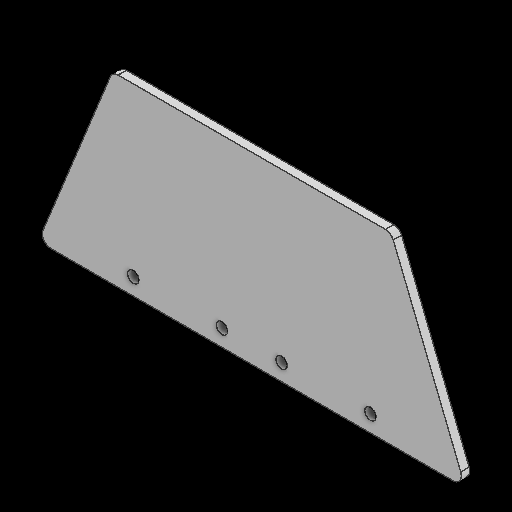
# Autodesk Inventor part: BreakerMount
Saved by Autodesk Inventor 2025.2 (Build 292293000, 293)
## iProperties
Created: 2025-11-18
Part Number: BreakerMount
Material: Generic
Document SubType Name: Sheet Metal
Designer: valer
Density: 1 g/cm^3
Sheet Metal Rule: Default
Appearance: Default
Author: valer
Autodesk Inventor part; units mm, degrees
ref_plane "YZ Plane" through (0, 0, 0) normal (1, 0, 0) x (0, 1, 0)
ref_plane "XZ Plane" through (0, 0, 0) normal (0, 1, 0) x (-1, 0, 0)
ref_plane "XY Plane" through (0, 0, 0) normal (0, 0, 1) x (1, 0, 0)
sketch "Base" plane through (0, 0, 0) normal (0, 0, 1) x (1, 0, 0)
  line L0 (0, 0) -> (70.3402, 0)
  line L1 (70.3402, 0) -> (115.4849, -88)
  line L2 (115.4849, -88) -> (0, -88)
  line L3 (0, -88) -> (0, 0) construction
  line L4 (0, 0) -> (-70.3402, 0)
  line L5 (-70.3402, 0) -> (-115.4849, -88)
  line L6 (-115.4849, -88) -> (0, -88)
  line L7 (-63.3831, 22.3248) -> (-182.4251, -209.7225) construction
  dimension "d1" = 88
  dimension "d3" = 4
  measures "d1" distance between parallel lines of L6 L4
  measures "d3" distance between parallel lines of L7 L5
extrude "Plate1" add sketch "Base" along normal blind 4
fillet "FilletsFeature" radius 6 4 edges at (-70.3402, 0, 2) (70.3402, 0, 2) (115.4849, -88, 2) (-115.4849, -88, 2)
sketch "BreakerMounts" plane through (0, 0, 0) normal (0, 0, -1) x (-1, 0, 0)
  circle A0 centre (56.75, -80) radius 2.75 projected
  circle A1 centre (14.25, -80) radius 2.75 projected
  circle A2 centre (-14.25, -80) radius 2.75 projected
  circle A3 centre (-56.75, -80) radius 2.75 projected
  point P0 (0, 0)
extrude "BreakerMountsFeature" cut sketch "BreakerMounts" against normal blind 4
sketch "FrameMounts" plane through (0, 0, 0) normal (0, 0, -1) x (-1, 0, 0)
  circle A0 centre (100.2396, -78) radius 3
  circle A1 centre (75.1349, -29.0638) radius 3
  line L0 (100.2396, -78) -> (75.1349, -29.0638) construction
  line L1 (72.0133, -3.2613) -> (111.0019, -79.2613) construction
  line L2 (105.6634, -88) -> (-105.6634, -88) projected
  line L3 (0, -105.6) -> (0, 17.6) construction
  circle A2 centre (-100.2396, -78) radius 3
  circle A3 centre (-75.1349, -29.0638) radius 3
  point P0 (0, 0)
  dimension "d6" = 6
  dimension "d7" = 6
  dimension "d8" = 10
  dimension "d9" = 9
  dimension "d10" = 55
  constraints: 4 centre point, 2 end point, 2 symmetric about line, 1 parallel, 2 other
  measures "d6" diameter of A0
  measures "d7" diameter of A1
  measures "d8" distance from line of L2 L0.start
  measures "d9" distance between parallel lines of L1 L0
  measures "d10" distance of L0.start L0.end
feature "FrameMountsFeature" [suppressed]
sketch "MatchProduction" plane through (0, 0, 4) normal (0, 0, 1) x (1, 0, 0)
  line L0 (0, -105.6) -> (0, 17.6) construction
  line L1 (-66.6748, 0) -> (66.6748, 0) projected
  line L2 (66.6748, 0) -> (102.2291, -88)
  line L3 (105.6634, -88) -> (-105.6634, -88) projected
  arc A0 (72.0133, -3.2613) -> (66.6748, 0) centre (66.6748, -6) ccw projected
  line L4 (72.0133, -3.2613) -> (111.0019, -79.2613) projected
  arc A1 (105.6634, -88) -> (111.0019, -79.2613) centre (105.6634, -82) ccw projected
  arc A2 (-111.0019, -79.2613) -> (-105.6634, -88) centre (-105.6634, -82) ccw projected
  line L5 (-111.0019, -79.2613) -> (-72.0133, -3.2613) projected
  arc A3 (-66.6748, 0) -> (-72.0133, -3.2613) centre (-66.6748, -6) ccw projected
  line L6 (-66.6748, 0) -> (-102.2291, -88)
  point P0 (0, 0)
  dimension "d13" = 68
  constraints: 4 end point, 1 point on line, 1 symmetric about line
  measures "d13" angle of L3 L2
extrude "MatchProductionFeature" cut sketch "MatchProduction" against normal blind 4 contours L6 L3 A2 L5 A3 | A0 L4 A1 L3 L2
fillet "Fillet2" radius 4 4 edges at (-102.2291, -88, 2) (102.2291, -88, 2) (66.6748, 0, 2) (-66.6748, 0, 2)
equation "\"d4\" = Thickness"
equation "\"d11\" = Thickness"
equation "\"d14\" = Thickness"
equation "\"d0\" = Thickness"
equation "\"BendRadius\" = Thickness"
equation "\"BendReliefWidth\" = Thickness"
equation "\"BendReliefDepth\" = 0.5 * Thickness"
equation "\"CornerReliefSize\" = 4 * Thickness"
equation "\"MinimumRemnant\" = 2 * Thickness"
equation "\"TransitionRadius\" = BendRadius"
equation "\"JacobiRadiusSize\" = BendRadius"
equation "\"GapSize\" = Thickness"
equation "\"Thickness\" = 4"
body "Solid1"
